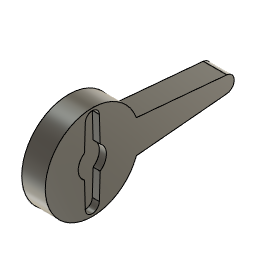
PinzaEscalada v1 v2 (Autodesk Fusion 360 design; units mm, degrees)
Autodesk Fusion 360 part; units mm, degrees
sketch "Boceto1" plane through (0, 0, 0) normal (1, 0, 0) x (0, 1, 0)
  arc A0 (85.8417, 2.5) -> (85.8417, -2.5) centre (87.5, 0) ccw
  arc A1 (89.1583, -2.5) -> (89.1583, 2.5) centre (87.5, 0) ccw
  line L0 (96.862, 3.505) -> (116.0692, 1.7779)
  line L1 (96.873, -3.4951) -> (116.0747, -1.7075)
  line L2 (85.8417, 2.5) -> (86.0006, 8.0231)
  line L3 (89.1583, 2.5) -> (88.9994, 8.0231)
  line L4 (85.8417, -2.5) -> (86.0006, -8.0231)
  line L5 (89.1583, -2.5) -> (88.9994, -8.0231)
  arc A2 (88.9994, 8.0231) -> (86.0006, 8.0231) centre (87.5, 7.98) ccw
  arc A3 (86.0006, -8.0231) -> (88.9994, -8.0231) centre (87.5, -7.98) ccw
  arc A4 (96.862, 3.505) -> (96.873, -3.4951) centre (87.5, -0.0098) ccw
  arc A5 (116.0747, -1.7075) -> (116.0692, 1.7779) centre (115.9125, 0.0349) ccw
  circle A6 centre (87.5, -0.0098) radius 2.5
  constraint coincident A1.start A0
  constraint concentric A0 A1
  constraint tangent L0 A5
  constraint tangent L1 A5
  constraint tangent L2 A2
  constraint tangent L3 A2
  constraint tangent L4 A3
  constraint tangent L5 A3
  constraint concentric A4 A6
extrude "Extruir5" add sketch "Boceto1" along normal blind 7 contours A0 A1 L2 L3 L4 L5 A2 A3 | A6 makes body 1
extrude "Extruir6" add sketch "Boceto1" along normal blind 10 contours L0 L1 A4 A5 bodies 1
sketch "Boceto2" plane through (0, 0, 0) normal (1, 0, 0) x (0, 1, 0)
extrude "Extruir7" add sketch "Boceto1" along normal blind 3.5 separate body contours A0 A1 L2 L3 L4 L5 A2 A3 | A6 makes body 2
extrude "Extruir8" add sketch "Boceto1" along normal blind 5 contours L0 L1 A4 A5 bodies 2
extrude "Extruir9" cut sketch "Boceto1" along normal blind 2.5 contours A6 bodies 2
scale "Escala1" factor 2 about (5, 96.862, 3.505) bodies 2
hidden bodies 1
